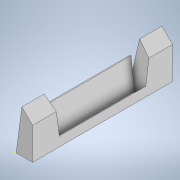
# Autodesk Inventor part: inside-join-half
Saved by Autodesk Inventor 2021 (Build 250183000, 183)
## iProperties
Created: 2020-12-10
Part Number: inside-join-half
Material: Generic
Document SubType Name: Modeling
Designer: Luke Kamols
Density: 1 g/cm^3
Appearance: Default
Author: Luke Kamols
Autodesk Inventor part; units mm, degrees
ref_plane "YZ Plane" through (0, 0, 0) normal (1, 0, 0) x (0, 1, 0)
ref_plane "XZ Plane" through (0, 0, 0) normal (0, 1, 0) x (-1, 0, 0)
ref_plane "XY Plane" through (0, 0, 0) normal (0, 0, 1) x (1, 0, 0)
sketch "Sketch1" plane through (0, 0, 0) normal (0, 0, 1) x (1, 0, 0)
  line L0 (0, 0) -> (6, 0)
  line L1 (6, 0) -> (6, 11)
  line L2 (6, 11) -> (2, 15)
  line L3 (2, 15) -> (0, 0)
  line L4 (0, 0) -> (0.4, 0)
  line L5 (0.4, 0) -> (2.3529, 14.6471)
  dimension "d0" = 6
  dimension "d3" = 11
  dimension "d38" = 0.4
  constraints: 12 end point, 2 point on line, 1 horizontal, 1 vertical
  measures "d0" distance of L0.start L0.end
  measures "d3" distance of L0.end L1.end
  measures "d38" distance of L0.start L4.end
extrude "Extrusion1" add sketch "Sketch1" along normal blind 9.6 contours L5 L2 L1 L0
sketch "Sketch2" plane through (0, 0, 9.6) normal (0, 0, 1) x (1, 0, 0)
  line L0 (0, 0) -> (6, 0) projected
  line L1 (0, 0) -> (3, 0)
  line L2 (2, 15) -> (0, 0) projected
  line L3 (0, 11) -> (3, 0)
  line L4 (0, 0) -> (-3, 0)
  line L5 (-3, 0) -> (0, 11)
  line L6 (6, 0) -> (6, 4)
  line L7 (6, 0) -> (6, 11) projected
  line L8 (6, 0) -> (5, 0)
  line L9 (5, 0) -> (6, 3.9744)
  line L10 (-3, 0) -> (-2.8, 0)
  line L11 (-2.8, 0) -> (0.1, 10.6333)
  line L12 (3, 0) -> (2.8, 0)
  line L13 (2.8, 0) -> (-0.1, 10.6333)
  line L14 (5, 0) -> (5.2, 0)
  line L15 (5.2, 0) -> (6, 3.1795)
  line L16 (2.8, 0) -> (2.6, 0)
  line L17 (2.6, 0) -> (0, 9.5333)
  line L18 (-2.8, 0) -> (-2.6, 0)
  line L19 (-2.6, 0) -> (0, 9.5333)
  line L20 (5.2, 0) -> (5.4, 0)
  line L21 (5.4, 0) -> (5.4, 0.7949)
  line L22 (0, 9.5333) -> (0, 8.9333)
  line L23 (0, 8.9333) -> (-0.1636, 8.9333)
  line L24 (0, 8.9333) -> (0.1636, 8.9333)
  point P0 (0, 10.2667)
  dimension "d6" = 3
  dimension "d7" = 11
  dimension "d8" = 3
  dimension "d27" = 4
  dimension "d28" = 1
  dimension "d29" = 0.2
  dimension "d30" = 0.2
  dimension "d31" = 0.2
  dimension "d44" = 0.2
  dimension "d45" = 0.2
  dimension "d48" = 0.2
  dimension "d49" = 0.6
  constraints: 44 end point, 15 point on line, 2 parallel, 2 perpendicular, 1 horizontal, 1 midpoint, 1 vertical
  measures "d6" distance of L0.start L1.end
  measures "d7" distance of L0.start L3.start
  measures "d8" distance of L0.start L4.end
  measures "d27" distance of L0.end L6.end
  measures "d28" distance of L0.end L8.end
  measures "d29" distance of L4.end L10.end
  measures "d30" distance of L1.end L12.end
  measures "d31" distance of L8.end L14.end
  measures "d44" distance of L12.end L16.end
  measures "d45" distance of L10.end L18.end
  measures "d48" distance of L14.end L20.end
  measures "d49" distance of L17.end L22.end
extrude "Extrusion2" add sketch "Sketch2" along normal blind 28.8 contours L2 L17 L0 | L4 L19 L23 L24 L17 L2 | L21 L15 L6 L0
sketch "Sketch3" plane through (0, 0, 38.4) normal (0, 0, 1) x (1, 0, 0)
  line L0 (6, 0) -> (6, 11) projected
  line L1 (0.4, 0) -> (6, 0) projected
  line L2 (6, 11) -> (2.3529, 14.6471) projected
  line L3 (2.3529, 14.6471) -> (0.4, 0) projected
  point P0 (0, 0)
extrude "Extrusion3" add sketch "Sketch3" along normal blind 9.6
sketch "Sketch4" plane through (6, 0, 0) normal (1, 0, 0) x (0, 0, -1)
  line L0 (-9.6, 11) -> (-9.6, 14.6471) projected
  line L1 (-9.6, 15) -> (-7.6, 15)
  line L2 (-9.6, 5.4179) -> (-9.6, 0) projected
  line L3 (-9.6, 15) -> (-9.6, 0)
  line L4 (-9.6, 0) -> (-7.6, 15)
  dimension "d40" = 2
  constraints: 6 end point, 1 collinear
  measures "d40" distance of L1.start L1.end
extrude "Extrusion4" cut sketch "Sketch4" against normal blind 23.3375
sketch "Sketch5" plane through (0, 0, 9.6) normal (0, 0, -1) x (-1, 0, 0)
  line L0 (2.6, 0) -> (-0.4, 0) projected
  line L1 (-5.2, 0) -> (-6, 3.1795) projected
  line L2 (-6, 0) -> (-6, 3.1795) projected
  line L3 (-5.2, 0) -> (-6, 0) projected
  line L4 (0.1636, 8.9333) -> (2.6, 0) projected
  line L5 (-0.1636, 8.9333) -> (-2.6, 0) projected
  line L6 (-2.6, 0) -> (-0.4, 0) projected
  line L7 (-0.1636, 8.9333) -> (0.1636, 8.9333) projected
extrude "Extrusion5" add sketch "Sketch5" along normal up to surface surface through (6, 15, 7.6) normal (0, -0.1321637, -0.9912279)
sketch "Sketch6" plane through (6, 0, 38.4) normal (1, 0, 0) x (0, 0, -1)
  line L0 (0, 8.9333) -> (0, 0) projected
  line L1 (0, 0) -> (0, 15)
  line L2 (0, 15) -> (-2, 15)
  line L3 (-2, 15) -> (0, 0)
  point P0 (38.4, 0)
  point P1 (0, 9.5333)
  dimension "d46" = 15
  dimension "d47" = 2
  constraints: 6 end point, 1 collinear, 1 perpendicular
  measures "d46" distance of L0.end L1.end
  measures "d47" distance of L1.end L2.end
extrude "Extrusion6" cut sketch "Sketch6" against normal blind 21.1125
sketch "Sketch7" plane through (0, 0, 38.4) normal (0, 0, 1) x (1, 0, 0)
  line L0 (2.6, 0) -> (0.1636, 8.9333) projected
  line L1 (-0.1636, 8.9333) -> (-2.6, 0) projected
  line L2 (-2.6, 0) -> (0.4, 0) projected
  line L3 (0.4, 0) -> (2.6, 0) projected
  line L4 (6, 3.1795) -> (5.4, 0.7949) projected
  line L5 (5.4, 0) -> (6, 0) projected
  line L6 (6, 3.1795) -> (6, 0) projected
  line L7 (5.4, 0.7949) -> (5.4, 0) projected
  line L8 (0.1636, 8.9333) -> (-0.1636, 8.9333) projected
extrude "Extrusion7" add sketch "Sketch7" against normal up to surface surface through (6, 0, 38.4) normal (0, -0.1321637, 0.9912279)
sketch "Sketch12" plane through (0, 0, 48) normal (0, 0, 1) x (1, 0, 0)
  point P0 (0, 0)
body "Solid1"
